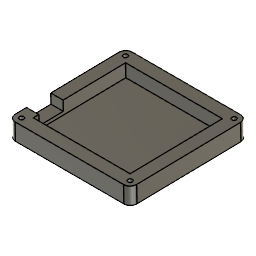
macropad fusion (Autodesk Fusion 360 design; units mm, degrees)
part number: 2026-06-24-19-05-01-669
Autodesk Fusion 360 part; units mm, degrees
note: some values were not read from the file. Chosen so that the rebuilt part matches the saved one: which bodies a step acts on; that a step has no effect.
form "Form1" [no effect]
sketch "sketch 210" plane through (0, 0, 0) normal (0, 1, 0) x (1, 0, 0)
  line L0 (0, 0) -> (74, 0)
  line L1 (74, 0) -> (74, -70.5)
  line L2 (74, -70.5) -> (0, -70.5)
  line L3 (0, -70.5) -> (0, 0)
  line L4 (-9.5, -80) -> (83.5, -80)
  line L5 (83.5, -80) -> (83.5, 9.5)
  line L6 (83.5, 9.5) -> (-9.5, 9.5)
  line L7 (-9.5, 9.5) -> (-9.5, -80)
  circle A0 centre (-4.5, 4.5) radius 1.7
  circle A1 centre (78.5, 4.5) radius 1.7
  circle A2 centre (78.5, -75) radius 1.7
  circle A3 centre (-4.5, -75) radius 1.7
  circle A4 centre (78.5, 4.5) radius 3
  circle A5 centre (-4.5, 4.5) radius 3
  circle A6 centre (-4.5, -75) radius 3
  circle A7 centre (78.5, -75) radius 3
  constraint horizontal L0
  constraint vertical L1
  constraint horizontal L2
  constraint vertical L3
  constraint coincident L0.start L3.end
  constraint horizontal L4
  constraint vertical L5
  constraint horizontal L6
  constraint vertical L7
  constraint concentric A1 A4
  constraint concentric A0 A5
  constraint concentric A3 A6
  constraint concentric A2 A7
extrude "Extrude1" add sketch "sketch 210" along normal blind 9.9 from surface at 3.1 contours A4 | A5 | A6 | A7 makes body 1 at (75.9401, 9.7, 76.5643) makes body 2 at (81.4963, 9.7, -4.3505) makes body 3 at (-1.6809, 9.7, 76.0261) makes body 4 at (-1.5037, 9.7, -4.3505)
extrude "Extrude2" add sketch "sketch 210" along normal blind 13 contours L4 L5 L6 L7 bodies 1 2 3 4
extrude "Extrude3" add sketch "sketch 210" along normal blind 3 contours L0 L1 L2 L3 bodies 1
sketch "Sketch1" plane through (0, 0, 0) normal (0, 1, 0) x (1, 0, 0)
sketch "Sketch3" plane through (0, 13, 0) normal (0, 1, 0) x (-1, 0, 0)
  circle A0 centre (-78.5, 75) radius 1.7
  circle A1 centre (4.5, -4.5) radius 1.7
  line L0 (-74, 70.5) -> (0, 70.5)
  line L1 (0, 70.5) -> (0, 0)
  line L2 (0, 0) -> (-74, 0)
  line L3 (-74, 0) -> (-74, 70.5)
  line L4 (9.5, -9.5) -> (9.5, 80)
  line L5 (9.5, 80) -> (-83.5, 80)
  line L6 (-83.5, 80) -> (-83.5, -9.5)
  line L7 (-83.5, -9.5) -> (9.5, -9.5)
  circle A2 centre (-78.5, -4.5) radius 1.7
  circle A3 centre (4.5, 75) radius 1.7
  line L8 (9.5, 66.25) -> (0, 66.25)
  line L9 (0, 66.25) -> (0, 47.75)
  line L10 (0, 47.75) -> (9.5, 47.75)
  line L11 (9.5, 47.75) -> (9.5, 66.25)
  line L12 (9.5, 80) -> (-83.5, 80)
  dimension "d10" = 18.5
  dimension "d11" = 13.75
  constraint horizontal L8
  constraint vertical L9
  constraint horizontal L10
  constraint vertical L11
  constraint coincident L4 L8.start
  measures "d10" distance of L8.start L10.end
  measures "d11" distance of L8 L12
extrude "Extrude4" cut sketch "Sketch3" against normal blind 7.5 contours L1 L4 L8 L9 L10 L11 bodies 1
move_body "Move1" bodies 1 to x (1, 0, 0) y (0, -0.017452, 0.999848) z (0, -0.999848, -0.017452) at (0, -9.4986, -9.6658)
fillet "Fillet1" radius 5 1 edges at (83.5, -89.5998, -4.563) on bodies 1
fillet "Fillet2" radius 5 1 edges at (83.5, -0.1134, -3.001) on bodies 1
fillet "Fillet3" radius 5 1 edges at (-9.5, -0.1134, -3.001) on bodies 1
fillet "Fillet4" radius 5 1 edges at (-9.5, -89.5998, -4.563) on bodies 1
